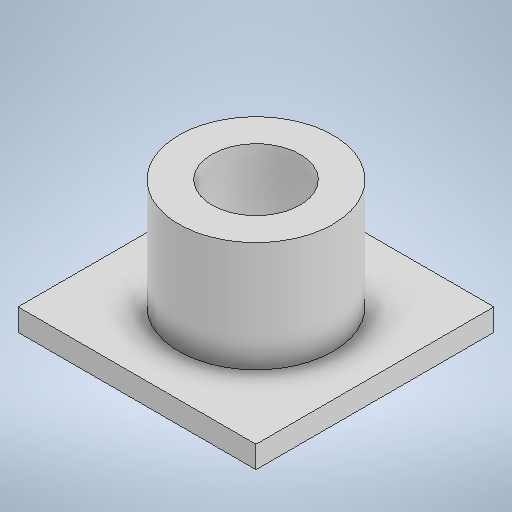
# Autodesk Inventor part: kapek
Saved by Autodesk Inventor 2025 (Build 290162000, 162)
## iProperties
Created: 2024-04-10
Part Number: kapek
Material: Ogólny
Document SubType Name: Modeling
Designer: user
Density: 1 g/cm^3
Appearance: Domyślna
Author: user
Autodesk Inventor part; units mm, degrees
ref_plane "YZ Plane" through (0, 0, 0) normal (1, 0, 0) x (0, 1, 0)
ref_plane "XZ Plane" through (0, 0, 0) normal (0, 1, 0) x (-1, 0, 0)
ref_plane "XY Plane" through (0, 0, 0) normal (0, 0, 1) x (1, 0, 0)
sketch "Szkic1" plane through (0, 0, 0) normal (0, 1, 0) x (-1, 0, 0)
  circle A0 centre (0, 0) radius 10
  line L0 (27, 0) -> (27, -27)
  line L1 (27, -27) -> (0, -27)
  line L2 (27, 0) -> (27, 27)
  line L3 (27, 27) -> (0, 27)
  line L4 (-27, 0) -> (-27, -27)
  line L5 (-27, -27) -> (0, -27)
  line L6 (-27, 0) -> (-27, 27)
  line L7 (-27, 27) -> (0, 27)
  circle A1 centre (0, 0) radius 17.5
  dimension "d0" = 20
  dimension "d6" = 54
  dimension "d7" = 54
  dimension "d8" = 35
  constraints: 16 end point, 2 centre point, 2 coincident
  measures "d0" diameter of A0
  measures "d6" distance between parallel lines of L6 L2
  measures "d7" distance between parallel lines of L1 L3
  measures "d8" diameter of A1
extrude "Wyciągnięcie proste1" add sketch "Szkic1" along normal blind 5
extrude "Wyciągnięcie proste2" add sketch "Szkic1" along normal blind 30 contours A1
